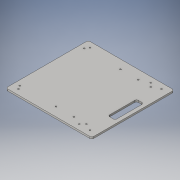
# Autodesk Inventor part: vrRig_v08_breadboardToSlideMount
Saved by Autodesk Inventor 2016 (Build 200138000, 138)
## iProperties
Created: 2018-03-27
Part Number: vrRig_v08_breadboardToSlideMount
Material: Generic
Document SubType Name: Modeling
Designer: harveylab
Density: 1 g/cm^3
Appearance: Default
Author: harveylab
Autodesk Inventor part; units mm, degrees
ref_plane "YZ Plane" through (0, 0, 0) normal (1, 0, 0) x (0, 1, 0)
ref_plane "XZ Plane" through (0, 0, 0) normal (0, 1, 0) x (-1, 0, 0)
ref_plane "XY Plane" through (0, 0, 0) normal (0, 0, 1) x (1, 0, 0)
sketch "Sketch1" plane through (0, 0, 0) normal (0, 1, 0) x (-1, 0, 0)
  line L0 (-304.8, 25.4) -> (-279.4, 25.4) construction
  line L1 (0, 25.4) -> (-25.4, 25.4) construction
  line L2 (0, 279.4) -> (-25.4, 279.4) construction
  line L3 (-304.8, 279.4) -> (-279.4, 279.4) construction
  circle A0 centre (-25.4, 279.4) radius 2.54
  circle A1 centre (-279.4, 279.4) radius 2.54
  circle A2 centre (-25.4, 25.4) radius 2.54
  circle A3 centre (-279.4, 25.4) radius 2.54
  line L4 (-304.8, 38.1) -> (-254, 38.1) construction
  circle A4 centre (-254, 38.1) radius 2.54
  line L5 (-304.8, 152.4) -> (-230.2081, 152.4) construction
  line L6 (-254, 38.1) -> (-209.55, 38.1) construction
  line L7 (-209.55, 38.1) -> (-146.05, 38.1) construction
  line L8 (-146.05, 38.1) -> (-17.526, 38.1) construction
  circle A5 centre (-209.55, 38.1) radius 2.54
  circle A6 centre (-146.05, 38.1) radius 2.54
  circle A7 centre (-17.526, 38.1) radius 2.54
  circle A8 centre (-254, 266.7) radius 2.54
  circle A9 centre (-209.55, 266.7) radius 2.54
  circle A10 centre (-146.05, 266.7) radius 2.54
  circle A11 centre (-17.526, 266.7) radius 2.54
  line L9 (-6.35, 298.45) -> (-298.45, 298.45)
  line L10 (-6.35, 6.35) -> (-298.45, 6.35)
  line L11 (0, 292.1) -> (0, 12.7)
  line L12 (-304.8, 12.7) -> (-304.8, 292.1)
  line L13 (-304.8, 152.4) -> (-292.1, 152.4)
  line L14 (-292.1, 152.4) -> (-292.1, 196.85)
  line L15 (-285.75, 203.2) -> (-273.05, 203.2)
  line L16 (-266.7, 196.85) -> (-266.7, 107.95)
  line L17 (-273.05, 101.6) -> (-285.75, 101.6)
  line L18 (-292.1, 107.95) -> (-292.1, 152.4)
  arc A12 (-285.75, 203.2) -> (-292.1, 196.85) centre (-285.75, 196.85) ccw
  arc A13 (-292.1, 107.95) -> (-285.75, 101.6) centre (-285.75, 107.95) ccw
  arc A14 (-273.05, 101.6) -> (-266.7, 107.95) centre (-273.05, 107.95) ccw
  arc A15 (-266.7, 196.85) -> (-273.05, 203.2) centre (-273.05, 196.85) ccw
  arc A16 (-304.8, 12.7) -> (-298.45, 6.35) centre (-298.45, 12.7) ccw
  arc A17 (-298.45, 298.45) -> (-304.8, 292.1) centre (-298.45, 292.1) ccw
  arc A18 (0, 292.1) -> (-6.35, 298.45) centre (-6.35, 292.1) ccw
  arc A19 (-6.35, 6.35) -> (0, 12.7) centre (-6.35, 12.7) ccw
  line L19 (-279.4, 25.4) -> (-241.3, 25.4) construction
  circle A20 centre (-241.3, 25.4) radius 2.54
  circle A21 centre (-241.3, 279.4) radius 2.54
  point P0 (0, 0)
  point P1 (-292.1, 203.2)
  point P2 (-266.7, 203.2)
  point P3 (-266.7, 101.6)
  point P4 (-292.1, 101.6)
  dimension "d3" = 25.4
  dimension "d5" = 25.4
  dimension "d7" = 25.4
  dimension "d9" = 25.4
  dimension "d10" = 5.08
  dimension "d11" = 5.08
  dimension "d12" = 5.08
  dimension "d13" = 5.08
  dimension "d15" = 50.8
  dimension "d16" = 5.08
  dimension "d18" = 44.45
  dimension "d19" = 63.5
  dimension "d20" = 128.524
  dimension "d21" = 5.08
  dimension "d22" = 5.08
  dimension "d23" = 5.08
  dimension "d27" = 50.8
  dimension "d28" = 25.4
  dimension "d29" = 101.6
  dimension "d31" = 6.35
  dimension "d32" = 6.35
  dimension "d33" = 6.35
  dimension "d34" = 6.35
  dimension "d35" = 6.35
  dimension "d38" = 38.1
  dimension "d39" = 5.08
  constraints: 40 end point, 22 centre point, 16 point on circle, 16 tangent, 10 point on line, 9 coincident, 5 symmetric about line, 4 perpendicular, 3 equal radius, 3 horizontal, 2 parallel, 2 vertical, 5 other
  measures "d3" distance of L0.start L0.end
  measures "d5" distance of L1.start L1.end
  measures "d7" distance of L2.start L2.end
  measures "d9" distance of L3.start L3.end
  measures "d10" diameter of A0
  measures "d11" diameter of A1
  measures "d12" diameter of A2
  measures "d13" diameter of A3
  measures "d15" distance of L4.start L4.end
  measures "d16" diameter of A4
  measures "d18" distance of L6.start L6.end
  measures "d19" distance of L6.end L7.end
  measures "d20" distance of L7.end L8.end
  measures "d21" diameter of A5
  measures "d22" diameter of A6
  measures "d23" diameter of A7
  measures "d27" distance of L13.end point (-292.1, 203.2)
  measures "d28" distance of point (-292.1, 203.2) point (-266.7, 203.2)
  measures "d29" distance of point (-266.7, 203.2) point (-266.7, 101.6)
  measures "d31" radius of A12
  measures "d32" radius of A13
  measures "d33" radius of A14
  measures "d34" radius of A15
  measures "d35" radius of A16
  measures "d38" distance of L19.start L19.end
  measures "d39" diameter of A20
extrude "Extrusion2" add sketch "Sketch1" along normal blind 6.35
body "Solid2"
